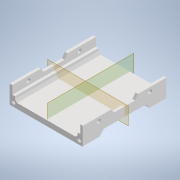
# Autodesk Inventor part: A-03
Saved by Autodesk Inventor 2022.2 (Build 262287000, 287)
## iProperties
Created: 2021-12-01
Part Number: A-03
Material: Generic
Document SubType Name: Modeling
Designer: kfcs7
Density: 1 g/cm^3
Appearance: Default
Author: kfcs7
Autodesk Inventor part; units mm, degrees
ref_plane "YZ Plane" through (0, 0, 0) normal (1, 0, 0) x (0, 1, 0)
ref_plane "XZ Plane" through (0, 0, 0) normal (0, 1, 0) x (-1, 0, 0)
ref_plane "XY Plane" through (0, 0, 0) normal (0, 0, 1) x (1, 0, 0)
sketch "Sketch1" plane through (0, 0, 0) normal (0, 1, 0) x (-1, 0, 0)
  line L0 (35, 40) -> (-35, 40)
  line L1 (-35, 40) -> (-35, -40)
  line L2 (-35, -40) -> (35, -40)
  line L3 (35, -40) -> (35, 40)
  line L4 (35, 40) -> (-35, -40) construction
  line L5 (-35, 40) -> (35, -40) construction
  point P0 (0, 0)
  dimension "d0" = 70
  dimension "d1" = 80
  constraints: 12 end point, 2 midpoint, 2 parallel, 1 horizontal, 1 perpendicular
  measures "d0" distance of L2.end L1.end
  measures "d1" distance of L1.end L0.end
extrude "Extrusion1" add sketch "Sketch1" along normal blind 17.5
chamfer "Chamfer1" distance 5 angle 45 2 edges at (35, 0, 0) (-35, 0, 0)
shell "Shell1" thickness 5 removed faces 3 at (10, 11.6667, 40) at (-10, 11.6667, -40) at (11.6667, 17.5, 13.3333)
ref_plane "Work Plane1" through (0, 17.5, -40) normal (-1, 0, 0) x (0, 0, 1)
ref_plane "Work Plane2" through (-30, 0, 0) normal (0, 0, 1) x (1, 0, 0)
sketch "Sketch10" plane through (-30, 0, 40) normal (0, 0, 1) x (1, 0, 0)
  line L0 (-5, 5) -> (-5, 17.5) projected
  line L1 (0, 0) -> (-5, 5) projected
  line L2 (0, 0) -> (60, 0) projected
  line L3 (65, 5) -> (60, 0) projected
  line L4 (65, 5) -> (65, 17.5) projected
  line L5 (60, 17.5) -> (65, 17.5) projected
  line L6 (60, 17.5) -> (60, 7.0711) projected
  line L7 (60, 7.0711) -> (57.9289, 5) projected
  line L8 (57.9289, 5) -> (2.0711, 5) projected
  line L9 (2.0711, 5) -> (0, 7.0711) projected
  line L10 (0, 7.0711) -> (0, 17.5) projected
  line L11 (-5, 17.5) -> (0, 17.5) projected
  line L12 (0, 0) -> (-5, 5) projected
  line L13 (-5, 5) -> (-5, 0)
  line L14 (-5, 0) -> (0, 0)
  point P0 (30, 0)
  constraints: 4 end point, 1 perpendicular, 1 point on line
extrude "Extrusion10" add sketch "Sketch10" against normal blind 20 contours L1 L14 L13
sketch "Sketch11" plane through (-35, 0, 40) normal (-1, 0, 0) x (0, 0, 1)
  line L0 (-80, 5) -> (-80, 17.5) projected
  line L1 (-20, 5) -> (-80, 5) projected
  line L2 (-20, 0) -> (-20, 5) projected
  line L3 (0, 0) -> (-20, 0) projected
  line L4 (0, 0) -> (0, 17.5) projected
  line L5 (-20, 0) -> (-20, 5) projected
  line L6 (-20, 5) -> (-15.8045, 0)
  line L7 (-20, 5) -> (-13.473, 5) construction
  line L8 (-80, 17.5) -> (0, 17.5) projected
  point P0 (-40, 0)
  point P1 (-15.8045, 0)
  dimension "d54" = 50
  constraints: 4 end point, 1 equal length, 1 horizontal
  measures "d54" angle of L6 L7
extrude "Extrusion11" cut sketch "Sketch11" against normal up to surface contours L6 L3 L2 surface through (-32.5, 2.5, -20) normal (-0.7071068, -0.7071068, 0)
sketch "Sketch12" plane through (-35, 0, 40) normal (0, 0, 1) x (1, 0, 0)
  line L0 (0, 0) -> (0, 17.5) projected
  line L1 (0, 0) -> (65, 0) projected
  line L2 (70, 5) -> (65, 0) projected
  line L3 (70, 5) -> (70, 17.5) projected
  line L4 (65, 17.5) -> (70, 17.5) projected
  line L5 (65, 17.5) -> (65, 7.0711) projected
  line L6 (65, 7.0711) -> (62.9289, 5) projected
  line L7 (62.9289, 5) -> (7.0711, 5) projected
  line L8 (7.0711, 5) -> (5, 7.0711) projected
  line L9 (5, 7.0711) -> (5, 17.5) projected
  line L10 (0, 17.5) -> (5, 17.5) projected
  line L11 (7.0711, 5) -> (5, 7.0711) projected
  line L12 (0, 0) -> (65, 0) projected
  line L13 (6.0355, 6.0355) -> (0, 0)
  circle A0 centre (3.5355, 3.5355) radius 1.25
  point P0 (35, 0)
  dimension "d57" = 5
  dimension "d58" = 2.5
  constraints: 2 end point, 1 centre point, 1 midpoint, 1 point on line
  measures "d57" distance of L0.start A0.centre
  measures "d58" diameter of A0
extrude "Extrusion12" cut sketch "Sketch12" against normal blind 5 draft 2.5 contours A0 L13 | L13 A0
mirror "Mirror3" about plane through (-30, 0, 0) normal (0, 0, 1) of "Extrusion12", "Extrusion11", "Extrusion10"
mirror "Mirror4" about plane through (0, 17.5, -40) normal (-1, 0, 0) of "Extrusion12", "Extrusion11", "Extrusion10", "Mirror3"
chamfer "Chamfer4" distance 0.5 angle 45 8 edges at (-32.7145, 3.5355, 40) (-35, 0, 32.0977) (32.7145, 3.5355, 40) (35, 0, 32.0977) (-35, 0, -32.0977) (-32.7145, 3.5355, -40) (32.7145, 3.5355, -40) (35, 0, -32.0977)
sketch "Sketch14" plane through (-35, 17.5, -40) normal (-1, 0, 0) x (0, 0, 1)
  circle A0 centre (64.5021, -4) radius 1.75 projected
  circle A1 centre (15.4979, -4) radius 1.75 projected
  point P0 (40, -17.5)
extrude "Extrusion14" cut sketch "Sketch14" against normal through all
sketch "Sketch15" plane through (-35, 17.5, -40) normal (-1, 0, 0) x (0, 0, 1)
  line L0 (0, 9) -> (16.2241, 9) projected
  line L1 (0, 9) -> (0, 0) projected
  line L2 (0, 0) -> (27.1992, 0) projected
  line L3 (27.1992, 0) -> (30, -4) projected
  line L4 (30, -4) -> (50, -4) projected
  line L5 (50, -4) -> (52.8008, 0) projected
  line L6 (52.8008, 0) -> (80, 0) projected
  line L7 (80, 9) -> (80, 0) projected
  line L8 (63.7759, 9) -> (80, 9) projected
  line L9 (63.7759, 9) -> (60, 4.5) projected
  line L10 (20, 4.5) -> (60, 4.5) projected
  line L11 (20, 4.5) -> (16.2241, 9) projected
  line L12 (52.8008, 0) -> (27.1992, 0)
  line L13 (80, 0) -> (0, 0) projected
  point P0 (40, -17.5)
  constraints: 2 end point, 1 collinear
extrude "Extrusion15" cut sketch "Sketch15" against normal blind 2.5 contours L12 L5 L4 L3
sketch "Sketch16" plane through (-30, 7.0711, -40) normal (1, 0, 0) x (0, 0, -1)
  line L0 (-61.2521, 2.6789) -> (-67.7521, 2.6789) construction
  line L1 (-68.2521, 3.1789) -> (-67.7521, 2.6789) construction
  line L2 (-68.2521, 3.1789) -> (-68.2521, 9.6789) construction
  line L3 (-67.7521, 10.1789) -> (-68.2521, 9.6789) construction
  line L4 (-67.7521, 10.1789) -> (-61.2521, 10.1789) construction
  line L5 (-60.7521, 9.6789) -> (-61.2521, 10.1789) construction
  line L6 (-60.7521, 9.6789) -> (-60.7521, 3.1789) construction
  line L7 (-61.2521, 2.6789) -> (-60.7521, 3.1789) construction
  line L8 (0, 12.8579) -> (-80, 12.8579) projected
  line L9 (-80, 2.4289) -> (-80, 12.8579) projected
  line L10 (0, 2.4289) -> (-80, 2.4289) projected
  line L11 (0, 12.8579) -> (0, 2.4289) projected
  line L12 (-12.2479, 2.6789) -> (-18.7479, 2.6789) construction
  line L13 (-19.2479, 3.1789) -> (-18.7479, 2.6789) construction
  line L14 (-19.2479, 3.1789) -> (-19.2479, 9.6789) construction
  line L15 (-18.7479, 10.1789) -> (-19.2479, 9.6789) construction
  line L16 (-18.7479, 10.1789) -> (-12.2479, 10.1789) construction
  line L17 (-11.7479, 9.6789) -> (-12.2479, 10.1789) construction
  line L18 (-11.7479, 9.6789) -> (-11.7479, 3.1789) construction
  line L19 (-12.2479, 2.6789) -> (-11.7479, 3.1789) construction
  point P0 (-40, -7.0711)
extrude "Extrusion16" cut sketch "Sketch16" against normal blind 2.5
mirror "Mirror5" about plane through (0, 17.5, -40) normal (-1, 0, 0) of "Extrusion16", "Extrusion15"
body "Solid1"
